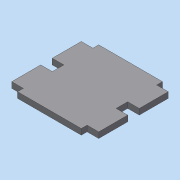
# Autodesk Inventor part: Motor-Side
Saved by Autodesk Inventor 2016 SP1 (Build 200210100, 210)
## iProperties
Created: 2016-03-02
Part Number: Motor-Side
Material: Generic
Document SubType Name: Modeling
Designer: Mohamed A.
Density: 1 g/cm^3
Appearance: Default
Author: Mohamed A.
Autodesk Inventor part; units mm, degrees
ref_plane "YZ Plane" through (0, 0, 0) normal (1, 0, 0) x (0, 1, 0)
ref_plane "XZ Plane" through (0, 0, 0) normal (0, 1, 0) x (-1, 0, 0)
ref_plane "XY Plane" through (0, 0, 0) normal (0, 0, 1) x (1, 0, 0)
sketch "Sketch2" plane through (0, 0, 0) normal (0, 0, 1) x (1, 0, 0)
  line L0 (16.5, 21) -> (-16.5, 21)
  line L1 (-16.5, 21) -> (-16.5, 18)
  line L2 (-16.5, -21) -> (16.5, -21)
  line L3 (16.5, -21) -> (16.5, -18)
  line L4 (-31.5, 0) -> (31.5, 0) construction
  line L5 (0, -29.4) -> (0, 29.4) construction
  line L6 (-16.5, 18) -> (-22.5, 18)
  line L7 (-22.5, 18) -> (-22.5, 3)
  line L8 (-22.5, 3) -> (-16.5, 3)
  line L9 (16.5, 18) -> (22.5, 18)
  line L10 (22.5, 18) -> (22.5, 3)
  line L11 (22.5, 3) -> (16.5, 3)
  line L12 (-16.5, -18) -> (-22.5, -18)
  line L13 (-22.5, -18) -> (-22.5, -3)
  line L14 (-22.5, -3) -> (-16.5, -3)
  line L15 (16.5, -18) -> (22.5, -18)
  line L16 (22.5, -18) -> (22.5, -3)
  line L17 (22.5, -3) -> (16.5, -3)
  line L18 (-16.5, 18) -> (-16.5, 3)
  line L19 (-16.5, 3) -> (-16.5, -3)
  line L20 (-16.5, -3) -> (-16.5, -18)
  line L21 (-16.5, -18) -> (-16.5, -21)
  line L22 (16.5, -3) -> (16.5, 3)
  line L23 (16.5, -18) -> (16.5, -3)
  line L24 (16.5, 3) -> (16.5, 18)
  line L25 (16.5, 18) -> (16.5, 21)
  point P0 (0, 0)
  dimension "d0" = 33
  dimension "d1" = 42
  dimension "d4" = 6
  dimension "d5" = 6
  dimension "d6" = 3
  dimension "d7" = 3
  constraints: 48 end point, 26 parallel, 12 perpendicular, 12 point on line, 8 symmetric about line, 2 horizontal, 2 other
  measures "d0" distance of L2.end L2.start
  measures "d1" distance of L2.start L0.end
  measures "d4" distance of L1.end L6.end
  measures "d5" distance of L9.start L9.end
  measures "d6" distance between parallel lines of L6 L0
  measures "d7" distance between parallel lines of L4 L8
extrude "Extrusion1" add sketch "Sketch2" along normal blind 3
body "Solid1"
